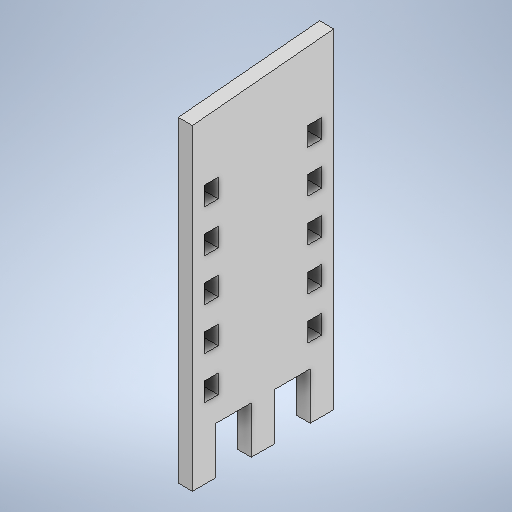
# Autodesk Inventor part: sort support wall 1
Saved by Autodesk Inventor 2025.3 (Build 293356000, 356)
## iProperties
Created: 2026-04-27
Part Number: sort support wall 1
Material: Generic
Document SubType Name: Modeling
Designer: kamal
Density: 1 g/cm^3
Appearance: Default
Author: kamal
Autodesk Inventor part; units mm, degrees
ref_plane "YZ Plane" through (0, 0, 0) normal (1, 0, 0) x (0, 1, 0)
ref_plane "XZ Plane" through (0, 0, 0) normal (0, 1, 0) x (-1, 0, 0)
ref_plane "XY Plane" through (0, 0, 0) normal (0, 0, 1) x (1, 0, 0)
sketch "Sketch1" plane through (0, 0, 0) normal (1, 0, 0) x (0, 1, 0)
  line L0 (0, 0) -> (120, 0)
  line L1 (0, 0) -> (0, 10) construction
  line L2 (0, 60) -> (114.4657, 60)
  line L3 (114.4657, 60) -> (120, 0)
  line L4 (0, 60) -> (-20, 60)
  line L5 (-20, 60) -> (-20, 50)
  line L6 (-20, 50) -> (0, 50)
  line L7 (0, 50) -> (0, 60) construction
  line L8 (0, 0) -> (-20, 0)
  line L9 (-20, 0) -> (-20, 10)
  line L10 (-20, 10) -> (0, 10)
  line L11 (0, 10) -> (0, 0) construction
  line L12 (0, 35) -> (-20, 35)
  line L13 (-20, 35) -> (-20, 25)
  line L14 (-20, 25) -> (0, 25)
  line L15 (0, 25) -> (0, 35) construction
  line L16 (0, 50) -> (0, 60) construction
  line L17 (0, 25) -> (0, 35) construction
  line L18 (0, 35) -> (0, 50)
  line L19 (0, 10) -> (0, 25)
  line L20 (90, 5) -> (82, 5)
  line L21 (82, 5) -> (82, 11)
  line L22 (82, 11) -> (90, 11)
  line L23 (90, 11) -> (90, 5)
  line L24 (72, 5) -> (64, 5)
  line L25 (64, 5) -> (64, 11)
  line L26 (64, 11) -> (72, 11)
  line L27 (72, 11) -> (72, 5)
  line L28 (54, 5) -> (46, 5)
  line L29 (46, 5) -> (46, 11)
  line L30 (46, 11) -> (54, 11)
  line L31 (54, 11) -> (54, 5)
  line L32 (36, 5) -> (28, 5)
  line L33 (28, 5) -> (28, 11)
  line L34 (28, 11) -> (36, 11)
  line L35 (36, 11) -> (36, 5)
  line L36 (18, 5) -> (10, 5)
  line L37 (10, 5) -> (10, 11)
  line L38 (10, 11) -> (18, 11)
  line L39 (18, 11) -> (18, 5)
  line L40 (90, 49) -> (82, 49)
  line L41 (82, 49) -> (82, 55)
  line L42 (82, 55) -> (90, 55)
  line L43 (90, 55) -> (90, 49)
  line L44 (64, 55) -> (72, 55)
  line L45 (72, 49) -> (64, 49)
  line L46 (72, 55) -> (72, 49)
  line L47 (64, 49) -> (64, 55)
  line L48 (46, 55) -> (54, 55)
  line L49 (54, 49) -> (46, 49)
  line L50 (54, 55) -> (54, 49)
  line L51 (46, 49) -> (46, 55)
  line L52 (28, 55) -> (36, 55)
  line L53 (36, 49) -> (28, 49)
  line L54 (36, 55) -> (36, 49)
  line L55 (28, 49) -> (28, 55)
  line L56 (10, 49) -> (10, 55)
  line L57 (10, 55) -> (18, 55)
  line L58 (18, 49) -> (10, 49)
  line L59 (18, 55) -> (18, 49)
  point P0 (-10, 35)
  point P1 (86, 5)
  point P2 (0, 5)
  point P3 (90, 8)
  point P4 (68, 5)
  point P5 (72, 8)
  point P6 (50, 5)
  point P7 (54, 8)
  point P8 (32, 5)
  point P9 (36, 8)
  point P10 (14, 5)
  point P11 (18, 8)
  point P12 (82, 8)
  point P13 (64, 8)
  point P14 (46, 8)
  point P15 (28, 8)
  point P16 (86, 49)
  point P17 (90, 52)
  point P18 (72, 52)
  point P19 (68, 49)
  point P20 (54, 52)
  point P21 (50, 49)
  point P22 (36, 52)
  point P23 (32, 49)
  point P24 (82, 52)
  point P25 (64, 52)
  point P26 (46, 52)
  point P27 (28, 52)
  point P28 (86, 55)
  point P29 (68, 55)
  point P30 (50, 55)
  point P31 (32, 55)
  point P32 (0, 30)
  point P33 (10, 52)
  point P34 (14, 49)
  point P35 (18, 52)
  point P36 (14, 55)
  dimension "d0" = 120
  dimension "d5" = 60
  dimension "d6" = 95.27
  dimension "d7" = 20
  dimension "d8" = 10
  dimension "d9" = 20
  dimension "d10" = 10
  dimension "d11" = 20
  dimension "d12" = 10
  dimension "d13" = 15
  dimension "d16" = 6
  dimension "d17" = 8
  dimension "d18" = 5
  dimension "d19" = 90
  dimension "d20" = 6
  dimension "d21" = 8
  dimension "d22" = 6
  dimension "d23" = 8
  dimension "d24" = 6
  dimension "d25" = 8
  dimension "d26" = 6
  dimension "d27" = 8
  dimension "d28" = 10
  dimension "d29" = 10
  dimension "d30" = 10
  dimension "d31" = 10
  dimension "d32" = 5
  dimension "d33" = 5
  dimension "d34" = 5
  dimension "d35" = 5
  dimension "d37" = 6
  dimension "d38" = 8
  dimension "d40" = 6
  dimension "d41" = 8
  dimension "d42" = 6
  dimension "d43" = 8
  dimension "d44" = 6
  dimension "d45" = 8
  dimension "d48" = 10
  dimension "d49" = 10
  dimension "d50" = 10
  dimension "d56" = 5
  dimension "d57" = 5
  dimension "d58" = 5
  dimension "d59" = 5
  dimension "d60" = 90
  dimension "d65" = 6
  dimension "d66" = 8
  dimension "d67" = 5
  dimension "d68" = 10
  constraints: 120 end point, 37 midpoint, 26 parallel, 18 perpendicular, 14 horizontal, 5 vertical, 1 point on line
  measures "d0" distance of L0.start L0.end
  measures "d5" distance of L0.start L2.start
  measures "d6" angle of L2 L3
  measures "d7" distance of L6.end L5.end
  measures "d8" distance of L5.end L4.end
  measures "d9" distance of L9.end L1.end
  measures "d10" distance of L8.end L9.end
  measures "d11" distance of L14.end L13.end
  measures "d12" distance of L13.end L12.end
  measures "d13" distance from line of L6 point (-10, 35)
  measures "d16" distance of L20.end L21.end
  measures "d17" distance of L21.end L22.end
  measures "d18" distance from line of L0 point (86, 5)
  measures "d19" horizontal distance of point (0, 5) point (90, 8)
  measures "d20" distance of L24.end L26.start
  measures "d21" distance of L26.start L26.end
  measures "d22" distance of L28.end L30.start
  measures "d23" distance of L30.start L30.end
  measures "d24" distance of L32.end L34.start
  measures "d25" distance of L34.start L34.end
  measures "d26" distance of L36.end L38.start
  measures "d27" distance of L38.start L38.end
  measures "d28" distance of point (72, 8) point (82, 8)
  measures "d29" distance of point (54, 8) point (64, 8)
  measures "d30" distance of point (36, 8) point (46, 8)
  measures "d31" distance of point (18, 8) point (28, 8)
  measures "d32" distance from line of L0 point (68, 5)
  measures "d33" distance between parallel lines of L0 L28
  measures "d34" distance from line of L0 point (32, 5)
  measures "d35" distance from line of L0 point (14, 5)
  measures "d37" distance of L41.start L41.end
  measures "d38" distance of L41.end L42.end
  measures "d40" distance of L47.start L47.end
  measures "d41" distance of L47.end L46.start
  measures "d42" distance of L49.end L51.end
  measures "d43" distance of L51.end L50.start
  measures "d44" distance of L55.start L55.end
  measures "d45" distance of L55.end L52.end
  measures "d48" distance of point (72, 52) point (82, 52)
  measures "d49" distance of point (54, 52) point (64, 52)
  measures "d50" distance of point (36, 52) point (46, 52)
  measures "d56" distance from line of L2 point (86, 55)
  measures "d57" distance from line of L2 point (68, 55)
  measures "d58" distance from line of L2 point (50, 55)
  measures "d59" distance from line of L2 point (32, 55)
  measures "d60" horizontal distance of point (0, 30) point (90, 52)
  measures "d65" distance of L58.end L56.end
  measures "d66" distance of L56.end L57.end
  measures "d67" distance between parallel lines of L2 L57
  measures "d68" distance of point (28, 52) point (18, 52)
extrude "Extrusion2" add sketch "Sketch1" along normal blind 6 contours L8 L9 L10 L19 L14 L13 L12 L18 L6 L5 L4 L2 L3 L0 | L20 L21 L22 L23 | L24 L25 L26 L27 | L28 L29 L30 L31 | L32 L33 L34 L35 | L36 L37 L38 L39 | L40 L41 L42 L43 | L44 L46 L45 L47 | L48 L50 L49 L51 | L52 L54 L53 L55 | L56 L57 L59 L58
extrude "Extrusion3" cut sketch "Sketch1" along normal blind 6 contours L20 L21 L22 L23 | L24 L25 L26 L27 | L28 L29 L30 L31 | L32 L33 L34 L35 | L36 L37 L38 L39 | L40 L41 L42 L43 | L44 L46 L45 L47 | L48 L50 L49 L51 | L52 L54 L53 L55 | L56 L57 L59 L58
body "Solid2"
